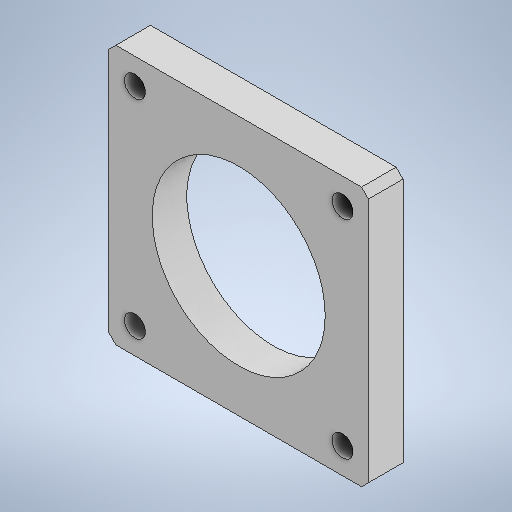
# Autodesk Inventor part: mst
Saved by Autodesk Inventor 2025.1 (Build 291241000, 241)
## iProperties
Created: 2024-11-12
Part Number: mst
Material: Ogólny
Document SubType Name: Modeling
Designer: PC
Density: 1 g/cm^3
Appearance: Domyślna
Author: PC
Autodesk Inventor part; units mm, degrees
ref_plane "YZ Plane" through (0, 0, 0) normal (1, 0, 0) x (0, 1, 0)
ref_plane "XZ Plane" through (0, 0, 0) normal (0, 1, 0) x (-1, 0, 0)
ref_plane "XY Plane" through (0, 0, 0) normal (0, 0, 1) x (1, 0, 0)
sketch "Szkic1" plane through (0, 0, 0) normal (0, 0, 1) x (1, 0, 0)
  line L0 (-30, 30) -> (30, 30) construction
  line L1 (30, 30) -> (30, -30) construction
  line L2 (30, -30) -> (-30, -30) construction
  line L3 (-30, -30) -> (-30, 30) construction
  line L4 (-30, 30) -> (30, -30) construction
  line L5 (30, 30) -> (-30, -30) construction
  circle A0 centre (-30, 30) radius 3.05
  circle A1 centre (-30, -30) radius 3.05
  circle A2 centre (30, -30) radius 3.05
  circle A3 centre (30, 30) radius 3.05
  line L6 (-35.5, 37.5) -> (35.5, 37.5)
  line L7 (37.5, 35.5) -> (37.5, -35.5)
  line L8 (35.5, -37.5) -> (-35.5, -37.5)
  line L9 (-37.5, -35.5) -> (-37.5, 35.5)
  line L10 (-37.5, 37.5) -> (37.5, -37.5) construction
  line L11 (37.5, 37.5) -> (-37.5, -37.5) construction
  line L12 (-37.5, 35.5) -> (-35.5, 37.5)
  line L13 (35.5, 37.5) -> (37.5, 35.5)
  line L14 (37.5, -35.5) -> (35.5, -37.5)
  line L15 (-37.5, -35.5) -> (-35.5, -37.5)
  circle A4 centre (0, 0) radius 25
  dimension "d0" = 60
  dimension "d1" = 60
  dimension "d2" = 6.1
  dimension "d3" = 75
  dimension "d4" = 75
  dimension "d5" = 2
  dimension "d6" = 2
  dimension "d7" = 2
  dimension "d8" = 2
  dimension "d9" = 2
  dimension "d10" = 2
  dimension "d11" = 2
  dimension "d12" = 2
  dimension "d13" = 50
  constraints: 32 end point, 8 point on line, 5 centre point, 5 coincident, 4 midpoint, 4 parallel, 3 equal radius, 2 horizontal, 2 perpendicular
  measures "d0" distance of L1.end L2.end
  measures "d1" distance of L0.end L1.end
  measures "d2" diameter of A0
  measures "d3" distance of L10.end L11.end
  measures "d4" distance of L11.start L10.end
  measures "d5" distance of L9.end L10.start
  measures "d6" distance of L6.start L10.start
  measures "d7" distance of L6.end L11.start
  measures "d8" distance of L7.start L11.start
  measures "d9" distance of L7.end L10.end
  measures "d10" distance of L8.start L10.end
  measures "d11" distance of L9.start L11.end
  measures "d12" distance of L8.end L11.end
  measures "d13" diameter of A4
extrude "Wyciągnięcie proste1" add sketch "Szkic1" along normal blind 10
equation "\"d6\" = d5"
equation "\"d7\" = d5"
equation "\"d8\" = d7"
equation "\"d9\" = d5"
equation "\"d10\" = d9"
equation "\"d11\" = d5"
equation "\"d12\" = d11"
